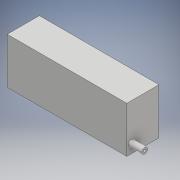
# Autodesk Inventor part: CajaDesague
Saved by Autodesk Inventor 2017 (Build 210142000, 142)
## iProperties
Created: 2021-08-26
Part Number: CajaDesague
Material: Generic
Document SubType Name: Modeling
Designer: USUARIO
Density: 1 g/cm^3
Appearance: Default
Author: USUARIO
Autodesk Inventor part; units mm, degrees
ref_plane "YZ Plane" through (0, 0, 0) normal (1, 0, 0) x (0, 1, 0)
ref_plane "XZ Plane" through (0, 0, 0) normal (0, 1, 0) x (-1, 0, 0)
ref_plane "XY Plane" through (0, 0, 0) normal (0, 0, 1) x (1, 0, 0)
sketch "Sketch1" plane through (0, 0, 0) normal (0, 1, 0) x (-1, 0, 0)
  line L0 (0, 0) -> (130, 0)
  line L1 (130, 0) -> (130, -50)
  line L2 (130, -50) -> (0, -50)
  line L3 (0, -50) -> (0, 0)
  dimension "d0" = 130
  dimension "d1" = 50
  constraints: 8 end point, 2 parallel, 1 horizontal, 1 perpendicular
  measures "d0" distance of L1.end L2.end
  measures "d1" distance of L0.end L1.end
extrude "Extrusion1" add sketch "Sketch1" along normal blind 1.27
sketch "Sketch2" plane through (0, 1.27, 0) normal (0, 1, 0) x (1, 0, 0)
  line L0 (-130, 0) -> (0, 0) projected
  line L1 (0, 0) -> (0, 50) projected
  line L2 (-130, 0) -> (0, 0)
  line L3 (0, 0) -> (0, 1.27)
  line L4 (0, 1.27) -> (-130, 1.27)
  line L5 (-130, 1.27) -> (-130, 0)
  line L6 (-130, 50) -> (-130, 0) projected
  line L7 (-130, 50) -> (0, 50)
  line L8 (0, 50) -> (0, 48.73)
  line L9 (0, 48.73) -> (-130, 48.73)
  line L10 (-130, 48.73) -> (-130, 50)
  line L11 (0, 1.27) -> (-1.27, 1.27)
  line L12 (-1.27, 1.27) -> (-1.27, 48.73)
  line L13 (-1.27, 48.73) -> (0, 48.73)
  line L14 (0, 48.73) -> (0, 1.27)
  line L15 (-130, 1.27) -> (-128.73, 1.27)
  line L16 (-128.73, 1.27) -> (-128.73, 48.73)
  line L17 (-128.73, 48.73) -> (-130, 48.73)
  line L18 (-130, 48.73) -> (-130, 1.27)
  dimension "d4" = 1.27
  dimension "d5" = 1.27
  dimension "d6" = 1.27
  dimension "d7" = 1.27
  constraints: 32 end point, 8 parallel, 4 horizontal, 4 perpendicular, 4 point on line
  measures "d4" distance of L3.end L2.end
  measures "d5" distance of L7.end L8.end
  measures "d6" distance of L12.end L13.end
  measures "d7" distance of L17.end L16.end
extrude "Extrusion2" add sketch "Sketch2" along normal blind 33.72 contours L5 L4 L1 L0 | L6 L9 L16 L4 | L4 L12 L9 L1 | L6 L7 L1 L9
sketch "Sketch3" plane through (0, 0, 0) normal (1, 0, 0) x (0, 0, -1)
  circle A0 centre (39.3882, 4.5) radius 3.175
  line L0 (50, 0) -> (0, 0) projected
  dimension "d10" = 6.35
  dimension "d17" = 4.5
  constraints: 1 centre point
  measures "d10" diameter of A0
  measures "d17" distance from line of L0 A0.centre
extrude "Extrusion3" add sketch "Sketch3" along normal blind 15
sketch "Sketch4" plane through (15, 4.5, -39.3882) normal (1, 0, 0) x (0, 0, -1)
  circle A0 centre (0, 0) radius 1.5
  point P0 (-39.3882, -4.5)
  dimension "d14" = 3
  constraints: 1 centre point
  measures "d14" diameter of A0
extrude "Extrusion4" cut sketch "Sketch4" against normal blind 30
body "Solid1"
